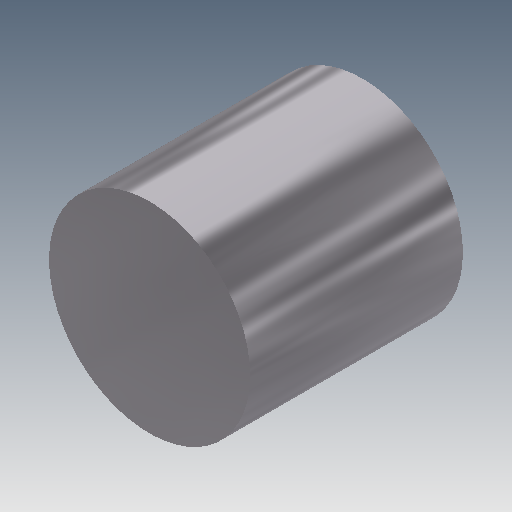
# Autodesk Inventor part: WeldExer_sleeve
Saved by Autodesk Inventor 2020.1 (Build 241239000, 239)
## iProperties
Part Number: WeldExer_sleeve
Document SubType Name: Modeling
Created: 2003-07-06
Designer: Ronald Myers
Manufacturer: Standard
Standards Organization: Custom
Stock Number: WeldExer_sleeve
Density: 1 g/cm^3
Material: Generic
Appearance: Aluminum (Polished)
Control State: 0
Master: False
Checked Out: False
Shininess: 64.0
Length Units: 11269
Angle Units: 11279
Time Units: 11290
Mass Units: 11286
Length Display Precision: 3
Angle Display Precision: 2
Compacted: True
Density: 0.0
Volumn: 0.0
Area: 0.0
PropertySet Name: Model Information
Author: Ronald Myers
Autodesk Inventor part; units mm, degrees
ref_plane "YZ Plane" through (0, 0, 0) normal (1, 0, 0) x (0, 1, 0)
ref_plane "XZ Plane" through (0, 0, 0) normal (0, 1, 0) x (-1, 0, 0)
ref_plane "XY Plane" through (0, 0, 0) normal (0, 0, 1) x (1, 0, 0)
sketch "Sketch1" plane through (0, 0, 0) normal (0, 0, 1) x (1, 0, 0)
  circle A0 centre (-3.3156, 2.0557) radius 8.5
  dimension "d0" = 17
  dimension "d0" = 17
  constraints: 1 centre point
  measures "d0" diameter of A0
extrude "Extrusion1" add sketch "Sketch1" against normal mid plane 18
body "Solid1"
